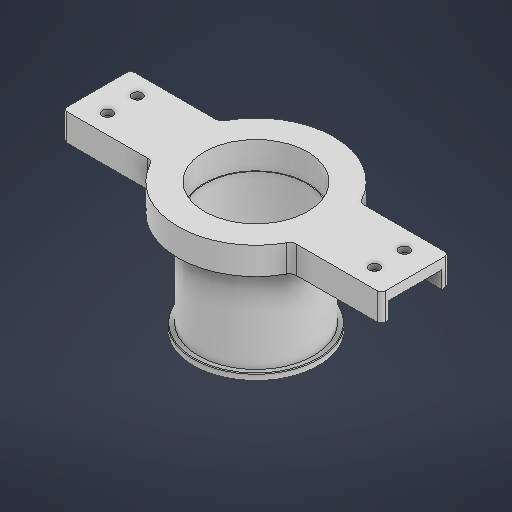
# Autodesk Inventor part: Cylinder  Segment - 11
Saved by Autodesk Inventor 2025 (Build 290162000, 162)
## iProperties
Created: 2024-04-11
Part Number: Cylinder  Segment - 11
Material: Generic
Document SubType Name: Modeling
Designer: Thienan Hoang
Density: 1 g/cm^3
Appearance: Default
Author: Thienan Hoang
Autodesk Inventor part; units mm, degrees
ref_plane "YZ Plane" through (0, 0, 0) normal (1, 0, 0) x (0, 1, 0)
ref_plane "XZ Plane" through (0, 0, 0) normal (0, 1, 0) x (-1, 0, 0)
ref_plane "XY Plane" through (0, 0, 0) normal (0, 0, 1) x (1, 0, 0)
sketch "Sketch1" plane through (0, 0, 0) normal (0, 1, 0) x (-1, 0, 0)
  circle A0 centre (0, 0) radius 46.125
  circle A1 centre (0, 0) radius 42.5
  circle A2 centre (0, 0) radius 37.5
  circle A3 centre (0, 0) radius 9.5
  dimension "Absolute_Diameter" = 92.25
  dimension "Diameter_No_Outer_Lip" = 85
  dimension "Inner_Cylinder_Diameter" = 75
  dimension "Lip_Diameter" = 19
  constraints: 4 centre point, 4 coincident
  measures "Absolute_Diameter" diameter of A0
  measures "Diameter_No_Outer_Lip" diameter of A1
  measures "Inner_Cylinder_Diameter" diameter of A2
  measures "Lip_Diameter" diameter of A3
extrude "Extrusion1" add sketch "Sketch1" along normal blind 5 contours A0
extrude "Extrusion2" add sketch "Sketch1" along normal blind 75 contours A1
sketch "Sketch2" plane through (0, 75, 0) normal (0, 1, 0) x (1, 0, 0)
  circle A0 centre (0, 0) radius 42.5
  dimension "Inner_Lip_Diameter" = 0
  dimension "Lip_Diameter_Out" = 85
  constraints: 1 centre point, 1 coincident, 2 other
  measures "Lip_Diameter_Out" diameter of A0
extrude "Extrusion7" [suppressed]
chamfer "Chamfer1" [suppressed]
chamfer "Chamfer2" distance 0.5 angle 45 3 edges at (46.125, 5, 0) (46.125, 0, 0) (37.5, 0, 0)
sketch "Sketch3" plane through (0, 5, 0) normal (0, 1, 0) x (1, 0, 0)
  circle A0 centre (0, 0) radius 127.5
  circle A1 centre (-127.5, 0) radius 2.5
  circle A2 centre (-103.1497, -74.9426) radius 2.5
  circle A3 centre (-39.3997, -121.2597) radius 2.5
  circle A4 centre (39.3997, -121.2597) radius 2.5
  circle A5 centre (103.1497, -74.9426) radius 2.5
  circle A6 centre (127.5, 0) radius 2.5
  circle A7 centre (103.1497, 74.9426) radius 2.5
  circle A8 centre (39.3997, 121.2597) radius 2.5
  circle A9 centre (-39.3997, 121.2597) radius 2.5
  circle A10 centre (-103.1497, 74.9426) radius 2.5
  dimension "d27" = 255
  dimension "d28" = 5
  dimension "d31" = 360
  constraints: 10 centre point, 1 coincident, 1 horizontal alignment, 23 other
  measures "d28" diameter of A1
extrude "Extrusion8" [suppressed]
sketch "Sketch6" plane through (0, 75, 0) normal (0, 1, 0) x (1, 0, 0)
  circle A0 centre (0, 0) radius 38.125
  line L0 (117.5, 25) -> (117.5, -25)
  line L1 (-117.5, -25) -> (-117.5, 25)
  arc A1 (-51.7808, -25) -> (51.7808, -25) centre (0, 0) ccw
  arc A2 (51.7808, 25) -> (-51.7808, 25) centre (0, 0) ccw
  line L2 (117.5, -25) -> (51.7808, -25)
  line L3 (-51.7808, -25) -> (-117.5, -25)
  line L4 (-117.5, 25) -> (-51.7808, 25)
  line L5 (51.7808, 25) -> (117.5, 25)
  dimension "d50" = 50
  dimension "d52" = 65.7192
  dimension "d53" = 76.25
  dimension "d54" = 57.5
  dimension "d55" = 57.5
  dimension "d56" = 50
  dimension "d57" = 235
  constraints: 12 end point, 5 parallel, 4 point on circle, 3 centre point, 2 coincident, 2 horizontal, 2 perpendicular
  measures "d50" distance of L0.start L0.end
  measures "d52" distance of L5.start L0.start
  measures "d53" diameter of A0
  measures "d54" radius of A2
  measures "d55" radius of A1
  measures "d56" distance of L1.start L1.end
  measures "d57" distance between parallel lines of L0 L1
extrude "Extrusion9" add sketch "Sketch6" along normal blind 20
fillet "Fillet1" radius 3 4 edges at (117.5, 85, 25) (117.5, 85, -25) (-117.5, 85, -25) (-117.5, 85, 25)
fillet "Fillet2" radius 5 4 edges at (-51.7808, 85, -25) (-51.7808, 85, 25) (51.7808, 85, -25) (51.7808, 85, 25)
sketch "Sketch7" plane through (0, 75, 0) normal (0, -1, 0) x (1, 0, 0)
  line L0 (117.25, -22) -> (-117.25, -22)
  line L1 (-117.25, -22) -> (-117.25, 22)
  line L2 (-117.25, 22) -> (117.25, 22)
  line L3 (117.25, 22) -> (117.25, -22)
  line L4 (117.25, -22) -> (-117.25, 22) construction
  line L5 (-117.25, -22) -> (117.25, 22) construction
  line L6 (145.5, -19.625) -> (92, -19.625)
  line L7 (89, -16.625) -> (89, 16.625)
  line L8 (92, 19.625) -> (145.5, 19.625)
  line L9 (145.5, 19.625) -> (145.5, -19.625)
  line L10 (145.5, -19.625) -> (89, 19.625) construction
  line L11 (89, -19.625) -> (145.5, 19.625) construction
  line L12 (-92, -19.625) -> (-145.5, -19.625)
  line L13 (-145.5, -19.625) -> (-145.5, 19.625)
  line L14 (-145.5, 19.625) -> (-92, 19.625)
  line L15 (-89, 16.625) -> (-89, -16.625)
  line L16 (-89, -19.625) -> (-145.5, 19.625) construction
  line L17 (-145.5, -19.625) -> (-89, 19.625) construction
  arc A0 (-92, -19.625) -> (-89, -16.625) centre (-92, -16.625) ccw
  arc A1 (-89, 16.625) -> (-92, 19.625) centre (-92, 16.625) ccw
  arc A2 (92, 19.625) -> (89, 16.625) centre (92, 16.625) ccw
  arc A3 (89, -16.625) -> (92, -19.625) centre (92, -16.625) ccw
  point P0 (0, 0)
  point P1 (117.25, 0)
  point P2 (-117.25, 0)
  dimension "d71" = 234.5
  dimension "d72" = 44
  dimension "d73" = 56.5
  dimension "d74" = 39.25
  dimension "d75" = 56.5
  dimension "d76" = 39.25
  dimension "d77" = 3
  dimension "d78" = 3
  constraints: 36 end point, 8 midpoint, 8 point on circle, 8 point on line, 8 tangent, 6 parallel, 4 centre point, 3 horizontal, 3 perpendicular, 2 equal radius
  measures "d71" distance of L1.end L2.end
  measures "d72" distance of L2.end L0.start
  measures "d73" distance of L10.end L8.end
  measures "d74" distance of L8.end L6.start
  measures "d75" distance of L13.end L17.end
  measures "d76" distance of L12.end L13.end
  measures "d77" radius of A0
  measures "d78" radius of A1
extrude "Extrusion10" cut sketch "Sketch7" against normal blind 12.575 contours L6 A3 L7 A2 L8 L3 | L3 L8 L9 L6 | L12 L13 L14 L1 | L1 L14 A1 L15 A0 L12
sketch "Sketch8" plane through (0, 87.575, 0) normal (0, -1, 0) x (1, 0, 0)
  line L0 (98.5, -11) -> (-98.5, -11)
  line L1 (-98.5, -11) -> (-98.5, 11)
  line L2 (-98.5, 11) -> (98.5, 11)
  line L3 (98.5, 11) -> (98.5, -11)
  line L4 (98.5, -11) -> (-98.5, 11) construction
  line L5 (-98.5, -11) -> (98.5, 11) construction
  circle A0 centre (98.5, -11) radius 2.5033
  circle A1 centre (98.5, 11) radius 3.8398
  circle A2 centre (-98.5, -11) radius 4.6851
  circle A3 centre (-98.5, 11) radius 7.9712
  point P0 (0, 0)
  dimension "d81" = 197
  dimension "d82" = 22
  constraints: 12 end point, 4 centre point, 4 coincident, 2 midpoint, 2 parallel, 1 horizontal, 1 perpendicular
  measures "d81" distance of L1.end L2.end
  measures "d82" distance of L0.end L1.end
hole "Hole2" at (98.5, 87.575, -11) at (98.5, 87.575, 11) at (-98.5, 87.575, -11) at (-98.5, 87.575, 11) direction (0, 1, 0) diameter 4.5 end through all
sketch "Sketch9" plane through (0, 95, 0) normal (0, 1, 0) x (1, 0, 0)
  circle A0 centre (98.5, -11) radius 2.25 projected
  circle A1 centre (98.5, -11) radius 3.75
  circle A2 centre (98.5, 11) radius 2.25 projected
  circle A3 centre (98.5, 11) radius 3.75
  circle A4 centre (-98.5, -11) radius 2.25 projected
  circle A5 centre (-98.5, -11) radius 3.75
  circle A6 centre (-98.5, 11) radius 2.25 projected
  circle A7 centre (-98.5, 11) radius 3.75
  point P0 (0, 0)
  dimension "d90" = 7.5
  dimension "d91" = 7.5
  dimension "d92" = 7.5
  constraints: 4 centre point, 4 coincident
  measures "d90" diameter of A1
  measures "d91" diameter of A3
  measures "d92" diameter of A5
extrude "Extrusion11" cut sketch "Sketch9" against normal blind 4.25 contours A0 | A1 | A2 | A3 | A4 | A5 | A6 | A7
body "Solid1"
